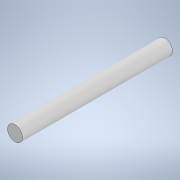
# Autodesk Inventor part: Pipe2
Saved by Autodesk Inventor 2021.3 (Build 253353010, 353A)
## iProperties
Created: 2021-07-13
Part Number: Pipe2
Material: Generic
Document SubType Name: Modeling
Designer: Dell
Density: 1 g/cm^3
Appearance: Default
Author: Dell
Autodesk Inventor part; units mm, degrees
ref_plane "YZ Plane" through (0, 0, 0) normal (1, 0, 0) x (0, 1, 0)
ref_plane "XZ Plane" through (0, 0, 0) normal (0, 1, 0) x (-1, 0, 0)
ref_plane "XY Plane" through (0, 0, 0) normal (0, 0, 1) x (1, 0, 0)
sketch "Sketch1" plane through (0, 0, 0) normal (0, 0, 1) x (1, 0, 0)
  circle A0 centre (-3.0143, 2.0313) radius 3.1746
  point P0 (0, 0)
  dimension "d0" = 63.5
  constraints: 1 centre point
extrude "Extrusion1" add sketch "Sketch1" along normal blind 63.5
body "Solid1"
